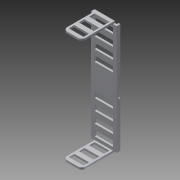
# Autodesk Inventor part: termination_lv_insulation
Saved by Autodesk Inventor 2014 SP1 (Build 180222100, 222)
## iProperties
Created: 2016-09-29
Part Number: termination_lv_insulation
Material: ABS Plastic
Document SubType Name: Modeling
Designer: tguillod
Density: 1.06 g/cm^3
Appearance: Smooth - White
Author: tguillod
Autodesk Inventor part; units mm, degrees
ref_plane "YZ Plane" through (0, 0, 0) normal (1, 0, 0) x (0, 1, 0)
ref_plane "XZ Plane" through (0, 0, 0) normal (0, 1, 0) x (-1, 0, 0)
ref_plane "XY Plane" through (0, 0, 0) normal (0, 0, 1) x (1, 0, 0)
sketch "Sketch1" plane through (0, 0, 0) normal (0, 0, 1) x (1, 0, 0)
  line L0 (0, 0) -> (10, 0)
  line L1 (10, 0) -> (10, 17)
  line L2 (10, 17) -> (0, 17)
  line L3 (0, 17) -> (0, 0)
  dimension "d0" = 17
  dimension "d1" = 10
  constraints: 8 end point, 2 parallel, 1 horizontal, 1 perpendicular
  measures "d0" distance of L0.end L1.end
  measures "d1" distance of L1.end L2.end
extrude "Extrusion1" add sketch "Sketch1" along normal blind 1
sketch "Sketch6" plane through (0, 0, 1) normal (0, 0, 1) x (1, 0, 0)
  line L0 (10, 0) -> (10, 17) projected
  line L1 (0, 17) -> (0, 0) projected
  line L2 (-2, 17) -> (12, 17)
  line L3 (12, 17) -> (12, 18)
  line L4 (12, 18) -> (-2, 18)
  line L5 (-2, 18) -> (-2, 17)
  dimension "d17" = 1
  dimension "d18" = 2
  dimension "d19" = 2
  constraints: 8 end point, 2 parallel, 1 horizontal, 1 perpendicular, 1 point on line
  measures "d17" distance of L2.end L3.end
  measures "d18" distance between parallel lines of L5 L1
  measures "d19" distance between parallel lines of L0 L3
extrude "Extrusion5" add sketch "Sketch6" against normal blind 25.75
sketch "Sketch7" plane through (-2, 18, 1) normal (0, 1, 0) x (1, 0, 0)
  line L0 (14, 0) -> (0, 0) projected
  line L1 (0, 25.75) -> (14, 25.75) projected
  line L2 (0, 0) -> (0, 25.75) projected
  line L3 (0, 0) -> (1, 0)
  line L4 (1, 0) -> (1, 25.75)
  line L5 (1, 25.75) -> (0, 25.75)
  line L6 (0, 25.75) -> (0, 0)
  line L7 (14, 25.75) -> (13, 25.75)
  line L8 (13, 25.75) -> (13, 0)
  line L9 (13, 0) -> (14, 0)
  line L10 (14, 0) -> (14, 25.75)
  line L11 (1, 25.75) -> (13, 25.75)
  line L12 (13, 25.75) -> (13, 24.75)
  line L13 (13, 24.75) -> (1, 24.75)
  line L14 (1, 24.75) -> (1, 25.75)
  point P0 (2, 1)
  dimension "d22" = 1
  dimension "d23" = 1
  dimension "d24" = 1
  constraints: 24 end point, 6 parallel, 3 horizontal, 3 perpendicular, 3 point on line
  measures "d22" distance between parallel lines of L10 L8
  measures "d23" distance between parallel lines of L2 L4
  measures "d24" distance between parallel lines of L1 L13
extrude "Extrusion6" add sketch "Sketch7" along normal blind 1 contours L0 L8 L1 L10 | L0 L2 L1 L4 | L13 L4 L1 L8
sketch "Sketch8" plane through (0, 0, -24.75) normal (0, 0, -1) x (-1, 0, 0)
  line L0 (-12, 17) -> (2, 17) projected
  line L1 (2, 17) -> (2, 19) projected
  line L2 (-12, 17) -> (2, 17)
  line L3 (2, 17) -> (2, 18)
  line L4 (2, 18) -> (-12, 18)
  line L5 (-12, 18) -> (-12, 17)
  point P0 (0, 0)
  dimension "d27" = 1
  constraints: 8 end point, 2 parallel, 1 horizontal, 1 midpoint, 1 perpendicular
  measures "d27" distance of L2.end L3.end
extrude "Extrusion7" add sketch "Sketch8" along normal blind 5
sketch "Sketch9" plane through (-1, 18, 1) normal (0, 1, 0) x (1, 0, 0)
  line L0 (0, 24.75) -> (0, 0) projected
  line L1 (12, 0) -> (12, 24.75) projected
  line L2 (12, 24.75) -> (0, 24.75) projected
  line L3 (1, 23.75) -> (11, 23.75)
  line L4 (11, 23.75) -> (11, 20.75)
  line L5 (11, 20.75) -> (1, 20.75)
  line L6 (1, 20.75) -> (1, 23.75)
  line L7 (1, 17.75) -> (11, 17.75)
  line L8 (11, 17.75) -> (11, 14.75)
  line L9 (11, 14.75) -> (1, 14.75)
  line L10 (1, 14.75) -> (1, 17.75)
  line L11 (1, 11.75) -> (11, 11.75)
  line L12 (11, 11.75) -> (11, 8.75)
  line L13 (11, 8.75) -> (1, 8.75)
  line L14 (1, 8.75) -> (1, 11.75)
  line L15 (1, 5.75) -> (11, 5.75)
  line L16 (11, 5.75) -> (11, 2.75)
  line L17 (11, 2.75) -> (1, 2.75)
  line L18 (1, 2.75) -> (1, 5.75)
  point P0 (1, 1)
  dimension "d30" = 1
  dimension "d31" = 1
  dimension "d32" = 3
  dimension "d33" = 3
  dimension "d34" = 1
  dimension "d35" = 3
  dimension "d36" = 3
  constraints: 32 end point, 9 collinear, 8 parallel, 4 horizontal, 4 perpendicular
  measures "d30" distance between parallel lines of L0 L6
  measures "d31" distance between parallel lines of L4 L1
  measures "d32" distance of L3.end L4.end
  measures "d33" distance between parallel lines of L5 L7
  measures "d34" distance between parallel lines of L2 L3
  measures "d35" distance between parallel lines of L9 L11
  measures "d36" distance between parallel lines of L13 L15
extrude "Extrusion8" cut sketch "Sketch9" against normal blind 3
sketch "Sketch10" plane through (0, 0, 1) normal (0, 0, 1) x (1, 0, 0)
  line L0 (0, 0) -> (10, 0) projected
  line L1 (10, 0) -> (10, 17) projected
  line L2 (0, 17) -> (0, 0) projected
  line L3 (1, 2) -> (9, 2)
  line L4 (9, 2) -> (9, 5)
  line L5 (9, 5) -> (1, 5)
  line L6 (1, 5) -> (1, 2)
  line L7 (9, 7.5) -> (1, 7.5)
  line L8 (1, 7.5) -> (1, 10.5)
  line L9 (1, 10.5) -> (9, 10.5)
  line L10 (9, 10.5) -> (9, 7.5)
  line L11 (1, 16) -> (9, 16)
  line L12 (9, 16) -> (9, 13)
  line L13 (9, 13) -> (1, 13)
  line L14 (1, 13) -> (1, 16)
  dimension "d39" = 1
  dimension "d40" = 1
  dimension "d41" = 2
  dimension "d42" = 2.5
  dimension "d43" = 2.5
  dimension "d44" = 3
  constraints: 24 end point, 6 collinear, 6 parallel, 3 horizontal, 3 perpendicular
  measures "d39" distance between parallel lines of L2 L6
  measures "d40" distance between parallel lines of L1 L4
  measures "d41" distance between parallel lines of L3 L0
  measures "d42" distance between parallel lines of L7 L5
  measures "d43" distance between parallel lines of L13 L9
  measures "d44" distance between parallel lines of L5 L3
extrude "Extrusion9" cut sketch "Sketch10" against normal blind 3
sketch "Sketch12" plane through (0, 0, 1) normal (0, 0, 1) x (1, 0, 0)
  line L0 (-2, 19) -> (-2, 17) projected
  line L1 (-2, 17) -> (0, 17) projected
  line L2 (-2, 19) -> (0, 19)
  line L3 (0, 19) -> (0, 17)
  line L4 (0, 17) -> (-2, 17)
  line L5 (-2, 17) -> (-2, 19)
  line L6 (12, 19) -> (10, 19)
  line L7 (10, 19) -> (10, 17)
  line L8 (10, 17) -> (12, 17)
  line L9 (12, 17) -> (12, 19)
  constraints: 16 end point, 4 parallel, 2 horizontal, 2 perpendicular
extrude "Extrusion10" cut sketch "Sketch12" against normal blind 1
mirror "Mirror1" about plane through (5, 17.5, -29.75) normal (0, 0, -1)
fillet "Fillet2" radius 2 4 edges at (0, 0, 0.5) (10, 0, 0.5) (10, 0, -60) (0, 0, -60)
body "Solid1"
